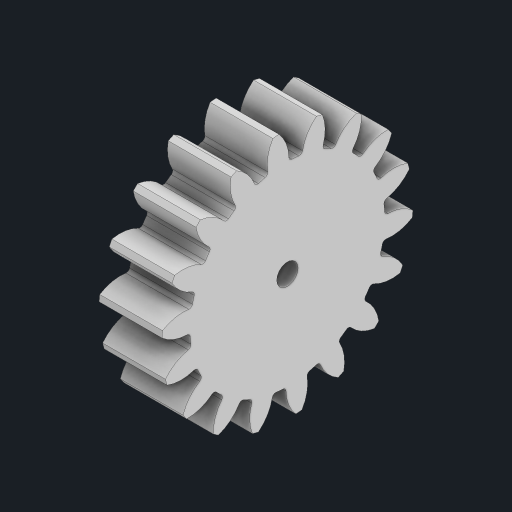
# Autodesk Inventor part: PINON DE TAPA PRINCIPAL
Saved by Autodesk Inventor 2024.3 (Build 283343000, 343)
## iProperties
Created: 2024-06-13
Part Number: PINON DE TAPA PRINCIPAL
Material: Generic
Document SubType Name: Modeling
Designer: Jhuliams
Density: 1 g/cm^3
Appearance: Default
Author: Jhuliams
Autodesk Inventor part; units mm, degrees
ref_plane "YZ Plane" through (0, 0, 0) normal (1, 0, 0) x (0, 1, 0)
ref_plane "XZ Plane" through (0, 0, 0) normal (0, 1, 0) x (-1, 0, 0)
ref_plane "XY Plane" through (0, 0, 0) normal (0, 0, 1) x (1, 0, 0)
sketch "Sketch1" plane through (0, 0, 0) normal (1, 0, 0) x (0, 1, 0)
  arc A0 (-3.216, -29.8271) -> (-1.751, -29.9489) centre (0, 0) ccw
  circle A1 centre (0, 0) radius 23.25
  line L0 (0, 0) -> (27, 0) construction
  arc A2 (-1.751, -29.9489) -> (0.5375, -23.2438) centre (-8.6776, -23.8416) ccw
  line L1 (0, 0) -> (27, 0) construction
  arc A3 (-4.3665, -22.8363) -> (-3.216, -29.8271) centre (4.6236, -24.9468) ccw
  arc A4 (3.7073, -22.9525) -> (7.1794, -29.1283) centre (12.8771, -21.861) ccw
  arc A5 (8.5977, -28.7416) -> (8.455, -21.6582) centre (0, -25.3717) ccw
  arc A6 (7.1794, -29.1283) -> (8.5977, -28.7416) centre (0, 0) ccw
  arc A7 (11.334, -20.3003) -> (16.7089, -24.9161) centre (19.5774, -16.1384) ccw
  arc A8 (17.9094, -24.0677) -> (15.3526, -17.4602) centre (8.6776, -23.8416) ccw
  arc A9 (16.7089, -24.9161) -> (17.9094, -24.0677) centre (0, 0) ccw
  arc A10 (17.5936, -15.1996) -> (24.223, -17.6987) centre (23.9164, -8.4692) ccw
  arc A11 (25.061, -16.4908) -> (20.3985, -11.1564) centre (16.3086, -19.4359) ccw
  arc A12 (24.223, -17.6987) -> (25.061, -16.4908) centre (0, 0) ccw
  arc A13 (21.7311, -8.2656) -> (28.8155, -8.3466) centre (25.3707, 0.2214) ccw
  arc A14 (29.1898, -6.925) -> (22.984, -3.5069) centre (21.9725, -12.6859) ccw
  arc A15 (28.8155, -8.3466) -> (29.1898, -6.925) centre (0, 0) ccw
  arc A16 (23.2476, -0.3347) -> (29.9324, 2.0123) centre (23.765, 8.8854) ccw
  arc A17 (29.7979, 3.4762) -> (22.7973, 4.5656) centre (24.9862, -4.4057) ccw
  arc A18 (29.9324, 2.0123) -> (29.7979, 3.4762) centre (0, 0) ccw
  arc A19 (21.9601, 7.6366) -> (27.439, 12.1284) centre (19.2928, 16.4776) ccw
  arc A20 (26.812, 13.458) -> (19.8609, 12.0874) centre (24.9862, 4.4057) ccw
  arc A21 (27.439, 12.1284) -> (26.812, 13.458) centre (0, 0) ccw
  arc A22 (18.0238, 14.6869) -> (21.6361, 20.7817) centre (12.4936, 22.0824) ccw
  arc A23 (20.5921, 21.8166) -> (14.529, 18.1513) centre (21.9725, 12.6859) ccw
  arc A24 (21.6361, 20.7817) -> (20.5921, 21.8166) centre (0, 0) ccw
  arc A25 (11.9136, 19.9657) -> (13.2235, 26.9284) centre (4.1875, 25.0237) ccw
  arc A26 (11.8885, 27.5438) -> (7.4447, 22.0259) centre (16.3086, 19.4359) ccw
  arc A27 (13.2235, 26.9284) -> (11.8885, 27.5438) centre (0, 0) ccw
  arc A28 (4.3665, 22.8363) -> (3.216, 29.8271) centre (-4.6236, 24.9468) ccw
  arc A29 (1.751, 29.9489) -> (-0.5375, 23.2438) centre (8.6776, 23.8416) ccw
  arc A30 (3.216, 29.8271) -> (1.751, 29.9489) centre (0, 0) ccw
  arc A31 (-3.7073, 22.9525) -> (-7.1794, 29.1283) centre (-12.8771, 21.861) ccw
  arc A32 (-8.5977, 28.7416) -> (-8.455, 21.6582) centre (0, 25.3717) ccw
  arc A33 (-7.1794, 29.1283) -> (-8.5977, 28.7416) centre (0, 0) ccw
  arc A34 (-11.334, 20.3003) -> (-16.7089, 24.9161) centre (-19.5774, 16.1384) ccw
  arc A35 (-17.9094, 24.0677) -> (-15.3526, 17.4602) centre (-8.6776, 23.8416) ccw
  arc A36 (-16.7089, 24.9161) -> (-17.9094, 24.0677) centre (0, 0) ccw
  arc A37 (-17.5936, 15.1996) -> (-24.223, 17.6987) centre (-23.9164, 8.4692) ccw
  arc A38 (-25.061, 16.4908) -> (-20.3985, 11.1564) centre (-16.3086, 19.4359) ccw
  arc A39 (-24.223, 17.6987) -> (-25.061, 16.4908) centre (0, 0) ccw
  arc A40 (-21.7311, 8.2656) -> (-28.8155, 8.3466) centre (-25.3707, -0.2214) ccw
  arc A41 (-29.1898, 6.925) -> (-22.984, 3.5069) centre (-21.9725, 12.6859) ccw
  arc A42 (-28.8155, 8.3466) -> (-29.1898, 6.925) centre (0, 0) ccw
  arc A43 (-23.2476, 0.3347) -> (-29.9324, -2.0123) centre (-23.765, -8.8854) ccw
  arc A44 (-29.7979, -3.4762) -> (-22.7973, -4.5656) centre (-24.9862, 4.4057) ccw
  arc A45 (-29.9324, -2.0123) -> (-29.7979, -3.4762) centre (0, 0) ccw
  arc A46 (-21.9601, -7.6366) -> (-27.439, -12.1284) centre (-19.2928, -16.4776) ccw
  arc A47 (-26.812, -13.458) -> (-19.8609, -12.0874) centre (-24.9862, -4.4057) ccw
  arc A48 (-27.439, -12.1284) -> (-26.812, -13.458) centre (0, 0) ccw
  arc A49 (-18.0238, -14.6869) -> (-21.6361, -20.7817) centre (-12.4936, -22.0824) ccw
  arc A50 (-20.5921, -21.8166) -> (-14.529, -18.1513) centre (-21.9725, -12.6859) ccw
  arc A51 (-21.6361, -20.7817) -> (-20.5921, -21.8166) centre (0, 0) ccw
  arc A52 (-11.9136, -19.9657) -> (-13.2235, -26.9284) centre (-4.1875, -25.0237) ccw
  arc A53 (-11.8885, -27.5438) -> (-7.4447, -22.0259) centre (-16.3086, -19.4359) ccw
  arc A54 (-13.2235, -26.9284) -> (-11.8885, -27.5438) centre (0, 0) ccw
  point P0 (14.529, 18.1513)
  point P1 (7.4447, 22.0259)
  point P2 (4.3665, 22.8363)
  point P3 (-0.5375, 23.2438)
  point P4 (-3.7073, 22.9525)
  point P5 (-11.334, 20.3003)
  point P6 (-15.3526, 17.4602)
  point P7 (-17.5936, 15.1996)
  point P8 (-22.984, 3.5069)
  point P9 (-23.2476, 0.3347)
  point P10 (-22.7973, -4.5656)
  point P11 (-21.9601, -7.6366)
  point P12 (-18.0238, -14.6869)
  point P13 (-14.529, -18.1513)
  point P14 (-7.4447, -22.0259)
  point P15 (-4.3665, -22.8363)
  point P16 (3.7073, -22.9525)
  point P17 (8.455, -21.6582)
  point P18 (11.334, -20.3003)
  point P19 (15.3526, -17.4602)
  point P20 (23.2476, -0.3347)
  point P21 (21.9601, 7.6366)
  point P22 (19.8609, 12.0874)
  dimension "d2" = 46.5
  dimension "d1" = 60
  dimension "d8" = 360
  constraints: 108 point on circle, 54 centre point, 4 end point, 2 horizontal, 1 coincident, 184 other
  measures "d1" diameter of A0
extrude "Extrusion1" add sketch "Sketch1" along normal blind 15
sketch "Sketch2" plane through (15, 0, 0) normal (1, 0, 0) x (0, 0, -1)
  circle A0 centre (0, 0) radius 2.55
  point P0 (-1.3836, 2.142)
  point P1 (1.3836, 2.142)
  point P2 (0, -2.55)
  dimension "d12" = 5.1
  constraints: 3 point on circle, 1 centre point, 1 coincident, 1 vertical alignment
  measures "d12" diameter of A0
extrude "Extrusion2" cut sketch "Sketch2" against normal blind 15
fillet "Fillet1" radius 0.78 2 edges at (7.5, 19.8609, 12.0874) (7.5, 18.0238, 14.6869)
pattern_circular "Circular Pattern1" count 18 over 360 about axis through (15, 0, 0) along (-1, 0, 0) of "Fillet1"
body "Solid1"
